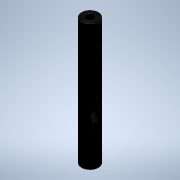
# Autodesk Inventor part: ABSスペーサーm3-45　簡易筒型
Saved by Autodesk Inventor 2020.2 (Build 242310000, 310)
## iProperties
Created: 2019-12-25
Part Number: ABSスペーサーm3-45　簡易筒型
Material: ABS プラスチック
Document SubType Name: Modeling
Designer: mozar
Density: 1.06 g/cm^3
Appearance: 滑らか - 黒
Mass: 0.449562 g
Surface Area: 6.07898 cm^2
Volume: 0.424115 cm^3
Author: mozar
Autodesk Inventor part; units mm, degrees
ref_plane "YZ Plane" through (0, 0, 0) normal (1, 0, 0) x (0, 1, 0)
ref_plane "XZ Plane" through (0, 0, 0) normal (0, 1, 0) x (-1, 0, 0)
sketch "スケッチ1" plane through (0, 0, 0) normal (0, 0, 1) x (1, 0, 0)
  circle A0 centre (0, 0) radius 3
  circle A1 centre (0, 0) radius 1.5
  dimension "d0" = 6
  dimension "d1" = 3
  constraints: 2 centre point, 2 coincident
  measures "d0" diameter of A0
  measures "d1" diameter of A1
extrude "押し出し1" add sketch "スケッチ1" along normal blind 45
ref_plane "作業平面1" through (0, 0, 39) normal (0, 0, 1) x (1, 0, 0)
sketch "スケッチ2" plane through (0, 0, 39) normal (0, 0, 1) x (1, 0, 0)
  point P0 (0, 0)
sketch "スケッチ3" plane through (0, 0, 39) normal (0, 0, 1) x (1, 0, 0)
  circle A0 centre (0, 0) radius 1.5 projected
  circle A1 centre (0, 0) radius 3 projected
extrude "押し出し2" add sketch "スケッチ3" against normal blind 33 contours A0
